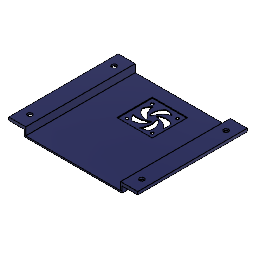
1-CBA bottom Cover V3 - part 1of3 v1 v12 (Autodesk Fusion 360 design; units mm, degrees)
Autodesk Fusion 360 part; units mm, degrees
note: some values were not read from the file. Set by a fixed rule: which sketch regions a step uses.
sketch "extrusion" plane through (0, 0, 0) normal (0, 1, 0) x (1, 0, 0)
  line L0 (-82.5, -8) -> (-62.5, -8)
  line L1 (-62.5, -8) -> (-62.5, 0)
  line L2 (-62.5, 0) -> (62.5, 0)
  line L3 (62.5, 0) -> (62.5, -8)
  line L4 (62.5, -8) -> (82.5, -8)
  line L5 (-60.5, -12) -> (-60.5, -2)
  line L6 (-60.5, -2) -> (60.5, -2)
  line L7 (60.5, -2) -> (60.5, -12)
  line L8 (-82.5, -12) -> (-60.5, -12)
  line L9 (60.5, -12) -> (82.5, -12)
  line L10 (-82.5, -8) -> (-82.5, -12)
  line L11 (82.5, -8) -> (82.5, -12)
  dimension "d1" = 125
  dimension "d2" = 8
  dimension "d3" = 20
  dimension "d4" = 8
  dimension "d5" = 20
  constraint horizontal L0
  constraint perpendicular L0 L1
  constraint perpendicular L1 L2
  constraint perpendicular L2 L3
  constraint perpendicular L1 L4
  constraint midpoint origin L2
  constraint parallel L1 L5
  constraint parallel L2 L6
  constraint parallel L3 L7
  constraint parallel L4 L9
  constraint parallel L0 L8
  constraint perpendicular L8 L10
  constraint perpendicular L9 L11
  measures "d1" distance of L1.end L2.end
  measures "d2" distance of L0.end L1.end
  measures "d3" distance of L0.start L0.end
  measures "d4" distance of L2.end L3.end
  measures "d5" distance of L3.end L4.end
extrude "Extrude1" add sketch "extrusion" along normal mid plane 140
sketch "top holes" plane through (0, 0, 12) normal (0, 0, 1) x (-1, 0, 0)
  circle A0 centre (71.5, -53.75) radius 3
  line L0 (82.5, -70) -> (60.5, -70)
  point P0 (71.5, -70)
  dimension "d11" = 6
  dimension "d12" = 16.25
  constraint midpoint L0 P0
  constraint vertical A0.centre P0
  measures "d11" diameter of A0
  measures "d12" distance of A0.centre L0
extrude "Extrude2" cut sketch "top holes" against normal blind 4
mirror "Mirror1" about plane through (0, 0, 0) normal (1, 0, 0) of "Extrude2"
mirror "Mirror2" about plane through (0, 0, 0) normal (0, 1, 0) of "Extrude2", "Mirror1"
sketch "square undent" plane through (0, 0, 2) normal (0, 0, 1) x (-1, 0, 0)
  line L0 (22.5, -53.5) -> (-22.5, -53.5)
  line L1 (-22.5, -53.5) -> (-22.5, -8.5)
  line L2 (-22.5, -8.5) -> (22.5, -8.5)
  line L3 (22.5, -8.5) -> (22.5, -53.5)
  line L4 (60.5, -70) -> (-60.5, -70)
  point P0 (0, -53.5)
  dimension "d17" = 45
  dimension "d18" = 45
  dimension "d19" = 16.5
  constraint horizontal L0
  constraint vertical L1
  constraint horizontal L2
  constraint vertical L3
  constraint midpoint L0 P0
  constraint vertical origin P0
  measures "d17" distance of L0.start L0.end
  measures "d18" distance of L0.start L2.end
  measures "d19" distance of L0.start L4
extrude "Extrude3" cut sketch "square undent" against normal blind 1
sketch "square holes" plane through (0, 0, 1) normal (0, 0, 1) x (-1, 0, 0)
  circle A0 centre (16.1, -47.1) radius 1.75
  line L0 (22.5, -53.5) -> (-22.5, -53.5)
  line L1 (22.5, -8.5) -> (22.5, -53.5)
  line L2 (-22.5, -8.5) -> (22.5, -53.5) construction
  circle A1 centre (0, -31) radius 18.5
  arc A2 (-18.1403, -27.3697) -> (-1.1682, -35.3966) centre (-1.8476, -14.8766) ccw
  arc A3 (-17.3688, -37.3697) -> (-0.6093, -37.262) centre (-9.0747, -23.9967) ccw
  arc A4 (-0.6093, -37.262) -> (-1.1682, -35.3966) centre (-1.1359, -36.4033) ccw
  point P0 (-22.5, -8.5)
  dimension "d22" = 3.5
  dimension "d23" = 6.4
  dimension "d24" = 6.4
  dimension "d25" = 37
  dimension "d47" = 10
  constraint coincident P0 L2.start
  constraint coincident L0.start L1.end
  constraint midpoint L2 A1.centre
  constraint coincident A1 A3.start
  constraint coincident A1 A2.start
  measures "d22" diameter of A0
  measures "d23" distance of A0.centre L0
  measures "d24" distance of A0.centre L1
  measures "d25" diameter of A1
  measures "d47" vertical distance of A2.start A3.start
extrude "Extrude4" cut sketch "square holes" against normal blind 1 contours A0
ref_plane "WorkPlane1" through (0, 31, 1.5) normal (0, -1, 0) x (-1, 0, 0)
mirror "Mirror3" about plane through (0, 31, 1.5) normal (0, -1, 0) of "Extrude4"
mirror "Mirror4" about plane through (0, 0, 0) normal (1, 0, 0) of "Extrude4", "Mirror3"
extrude "Extrude5" cut sketch "square holes" against normal blind 1 contours A1 A2 A3 A4 picked at (-15.1188, -35.3771)
pattern_circular "C-Pattern1" count 5 over 360 about axis through (0, 31, 1) along (0, 0, -1) of "Extrude5"
sketch "Sketch5" plane through (0, 0, 8) normal (0, 0, -1) x (1, 0, 0)
  circle A0 centre (71.5, 53.75) radius 3
  circle A1 centre (71.5, -53.75) radius 3
  line L0 (62.5, 70) -> (62.5, -70)
  line L1 (62.5, -70) -> (82.5, -70)
  line L2 (82.5, -70) -> (82.5, 70)
  line L3 (82.5, 70) -> (62.5, 70)
  circle A2 centre (71.5, -53.75) radius 5
  dimension "d35" = 10
  constraint concentric A1 A2
  measures "d35" diameter of A2
extrude "Extrude6" cut sketch "Sketch5" against normal blind 2 contours A2
sketch "Sketch6" plane through (0, 0, 8) normal (0, 0, -1) x (1, 0, 0)
  circle A0 centre (71.5, -53.75) radius 5
  circle A1 centre (71.5, 53.75) radius 3
  line L0 (62.5, 70) -> (62.5, -70)
  line L1 (62.5, -70) -> (82.5, -70)
  line L2 (82.5, -70) -> (82.5, 70)
  line L3 (82.5, 70) -> (62.5, 70)
  circle A2 centre (71.5, 53.75) radius 5
  dimension "d38" = 10
  constraint concentric A1 A2
  measures "d38" diameter of A2
extrude "Extrude7" cut sketch "Sketch6" against normal blind 2 contours A2
sketch "Sketch7" plane through (0, 0, 8) normal (0, 0, -1) x (1, 0, 0)
  circle A0 centre (-71.5, 53.75) radius 3
  circle A1 centre (-71.5, -53.75) radius 3
  line L0 (-82.5, 70) -> (-82.5, -70)
  line L1 (-82.5, -70) -> (-62.5, -70)
  line L2 (-62.5, -70) -> (-62.5, 70)
  line L3 (-62.5, 70) -> (-82.5, 70)
  circle A2 centre (-71.5, -53.75) radius 5
  dimension "d41" = 10
  constraint concentric A1 A2
  measures "d41" diameter of A2
extrude "Extrude8" cut sketch "Sketch7" against normal blind 2 contours A2
sketch "Sketch8" plane through (0, 0, 8) normal (0, 0, -1) x (1, 0, 0)
  circle A0 centre (-71.5, -53.75) radius 5
  circle A1 centre (-71.5, 53.75) radius 3
  line L0 (-82.5, 70) -> (-82.5, -70)
  line L1 (-82.5, -70) -> (-62.5, -70)
  line L2 (-62.5, -70) -> (-62.5, 70)
  line L3 (-62.5, 70) -> (-82.5, 70)
  circle A2 centre (-71.5, 53.75) radius 5
  dimension "d44" = 10
  constraint concentric A1 A2
  measures "d44" diameter of A2
extrude "Extrude9" cut sketch "Sketch8" against normal blind 2 contours A2
